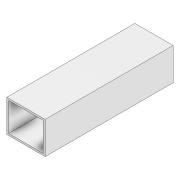
# Autodesk Inventor part: Cablecanal Ranurado 30x30 L=235 mm
Saved by Autodesk Inventor 2020 (Build 240168000, 168)
## iProperties
Created: 2020-07-11
Part Number: Cablecanal Ranurado 30x30 L=235 mm
Material: PPS Plastic
Document SubType Name: Modeling
Designer: Hernan
Density: 1.637 g/cm^3
Appearance: Smooth - White
Author: Hernan
Autodesk Inventor part; units mm, degrees
ref_plane "YZ Plane" through (0, 0, 0) normal (1, 0, 0) x (0, 1, 0)
ref_plane "XZ Plane" through (0, 0, 0) normal (0, 1, 0) x (-1, 0, 0)
ref_plane "XY Plane" through (0, 0, 0) normal (0, 0, 1) x (1, 0, 0)
sketch "Sketch1" plane through (0, 0, 0) normal (0, 0, 1) x (1, 0, 0)
  line L0 (-17.5599, -5.1941) -> (18.038, -5.1941)
  line L1 (18.038, -5.1941) -> (18.038, 24.8059)
  line L2 (18.038, 24.8059) -> (-17.5599, 24.8059)
  line L3 (-17.5599, 24.8059) -> (-17.5599, -5.1941)
  line L4 (-17.5599, 23.1059) -> (18.038, 23.1059)
  line L5 (16.338, 24.8059) -> (16.338, -5.1941)
  line L6 (-17.5599, -3.4941) -> (18.038, -3.4941)
  line L7 (-15.8599, -5.1941) -> (-15.8599, 24.8059)
  point P0 (0, 0)
  point P1 (-15.8599, 23.1059)
  point P2 (-15.8599, -3.4941)
  point P3 (16.338, -3.4941)
  point P4 (16.338, 23.1059)
  dimension "d0" = 30
  dimension "d1" = 1.7
  dimension "d2" = 1.7
  dimension "d3" = 1.7
  dimension "d4" = 1.7
  constraints: 16 end point, 8 point on line, 3 horizontal, 3 perpendicular, 2 vertical
  measures "d0" distance of L0.end L1.end
  measures "d1" distance between parallel lines of L7 L3
  measures "d2" distance between parallel lines of L2 L4
  measures "d3" distance between parallel lines of L1 L5
  measures "d4" distance between parallel lines of L0 L6
extrude "Extrusion1" add sketch "Sketch1" against normal blind 119.059
extrude "Extrusion2" cut sketch "Sketch1" against normal blind 235.08 contours L7 L4 L5 L6
body "Solid1"
